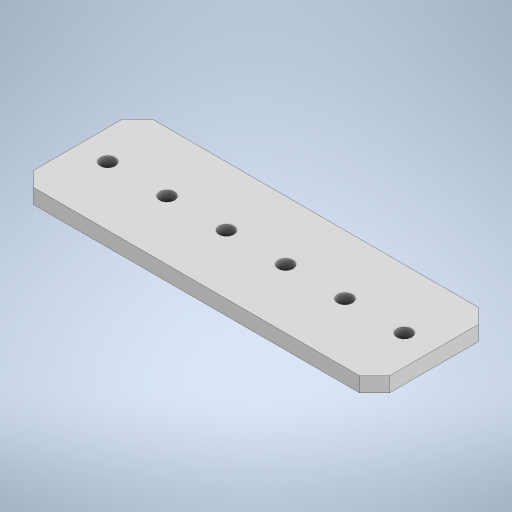
# Autodesk Inventor part: Straight Bracket (6)
Saved by Autodesk Inventor 2023 (Build 270158030, 158C)
## iProperties
Created: 2022-07-21
Part Number: Straight Bracket (6)
Material: Generic
Document SubType Name: Modeling
Designer: rm0990889
Density: 1 g/cm^3
Appearance: Default
Author: rm0990889
Autodesk Inventor part; units mm, degrees
ref_plane "YZ Plane" through (0, 0, 0) normal (1, 0, 0) x (0, 1, 0)
ref_plane "XZ Plane" through (0, 0, 0) normal (0, 1, 0) x (-1, 0, 0)
ref_plane "XY Plane" through (0, 0, 0) normal (0, 0, 1) x (1, 0, 0)
sketch "Sketch1" plane through (0, 0, 0) normal (0, 1, 0) x (-1, 0, 0)
  line L0 (0, 0) -> (11.2251, 0)
  circle A0 centre (6.35, -12.7) radius 1.5875
  circle A1 centre (19.05, -12.7) radius 1.5875
  circle A2 centre (31.75, -12.7) radius 1.5875
  circle A3 centre (44.45, -12.7) radius 1.5875
  circle A4 centre (57.15, -12.7) radius 1.5875
  circle A5 centre (69.85, -12.7) radius 1.5875
  line L1 (0, 0) -> (0, -22.225)
  line L2 (3.175, -25.4) -> (73.025, -25.4)
  line L3 (76.2, -22.225) -> (76.2, -3.175)
  line L4 (73.025, 0) -> (11.2251, 0)
  line L5 (73.025, 0) -> (76.2, -3.175)
  line L6 (76.2, -22.225) -> (73.025, -25.4)
  line L7 (3.175, -25.4) -> (0, -22.225)
  line L8 (3.175, 0) -> (0, -3.175)
  point P0 (5.6126, 0)
  point P1 (0, -25.4)
  point P2 (76.2, -25.4)
  point P3 (76.2, 0)
  dimension "d0" = 3.175
  dimension "d2" = 12.7
  dimension "d5" = 12.7
  dimension "d10" = 25.4
  dimension "d11" = 6.35
  dimension "d12" = 3.175
  dimension "d13" = 3.175
  dimension "d14" = 3.175
  dimension "d15" = 3.175
  dimension "d16" = 3.175
  dimension "d17" = 3.175
  constraints: 18 end point, 8 point on line, 6 centre point, 3 horizontal, 3 perpendicular, 1 midpoint, 1 vertical, 10 other
  measures "d0" diameter of A0
  measures "d2" vertical distance of A0.centre point (5.613, 0)
  measures "d5" distance of A0.centre A1.centre
  measures "d10" distance of L0.start point (0, -25.4)
  measures "d11" distance from line of L3 A5.centre
  measures "d12" distance of L4.start point (76.2, 0)
  measures "d13" distance of L3.end point (76.2, 0)
  measures "d14" distance of L3.start point (76.2, -25.4)
  measures "d15" distance of L2.end point (76.2, -25.4)
  measures "d16" distance of L2.start point (0, -25.4)
  measures "d17" distance of L1.end point (0, -25.4)
extrude "Extrusion1" add sketch "Sketch1" along normal blind 3.175 contours L0 L4 L5 L3 L6 L2 L7 L1 L8
equation "\"d13\" = d12"
equation "\"d14\" = d12"
equation "\"d15\" = d14"
equation "\"d16\" = d12"
equation "\"d17\" = d16"
body "Solid1"
